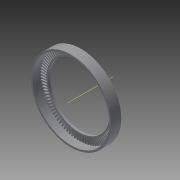
# Autodesk Inventor part: otackomer_new
Saved by Autodesk Inventor 2013 (Build 170138000, 138)
## iProperties
Created: 2015-05-28
Part Number: otackomer_new
Material: Generic
Document SubType Name: Modeling
Designer: Jufo
Density: 1 g/cm^3
Author: Jufo
Autodesk Inventor part; units mm, degrees
ref_plane "YZ Plane" through (0, 0, 0) normal (1, 0, 0) x (0, 1, 0)
ref_plane "XZ Plane" through (0, 0, 0) normal (0, 1, 0) x (-1, 0, 0)
ref_plane "XY Plane" through (0, 0, 0) normal (0, 0, 1) x (1, 0, 0)
sketch "Sketch1" plane through (0, 0, 0) normal (0, 1, 0) x (-1, 0, 0)
  circle A0 centre (0, 0) radius 28
  circle A1 centre (0, 0) radius 26.75
  dimension "d0" = 56
  dimension "d1" = 53.5
  constraints: 2 centre point, 2 coincident
  measures "d0" diameter of A0
  measures "d1" diameter of A1
extrude "Extrusion1" add sketch "Sketch1" along normal blind 7
sketch "Sketch2" plane through (0, 7, 0) normal (0, 1, 0) x (1, 0, 0)
  circle A0 centre (0, 0) radius 26.75 projected
  circle A1 centre (0, 0) radius 28 projected
  circle A2 centre (0, 0) radius 21.5
  circle A3 centre (0, 0) radius 22.5
  dimension "d4" = 43
  dimension "d5" = 45
  dimension "d6" = 1.25
  constraints: 2 centre point, 2 coincident
  measures "d4" diameter of A2
  measures "d5" diameter of A3
  measures "d6" radial gap between concentric circles of A1 A0
extrude "Extrusion2" add sketch "Sketch2" against normal blind 1.6 contours A3
sketch "Sketch3" plane through (0, 7, 0) normal (0, 1, 0) x (1, 0, 0)
  circle A0 centre (0, 0) radius 26.75 projected
  circle A1 centre (0, 0) radius 28 projected
  line L0 (0, 0) -> (8.005, 26.8313)
  line L1 (0, 0) -> (8.8439, 26.5666)
  line L2 (6.3306, 21.2189) -> (6.9905, 20.9992)
  line L3 (7.6477, 25.6335) -> (8.4491, 25.3806)
  dimension "d9" = 1.8
  constraints: 8 end point, 4 point on circle, 4 point on line, 1 perpendicular
  measures "d9" angle of L0 L1
extrude "Extrusion3" add sketch "Sketch3" against normal blind 1.6 contours L1 L2 L0 L3
pattern_circular "Circular Pattern1" count 90 over 360 about axis through (0, 0, 0) along (0, 1, 0) of "Extrusion3"
body "Solid1"
